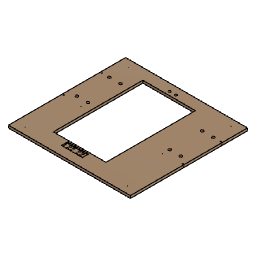
Underbase (Autodesk Fusion 360 design; units mm, degrees)
Autodesk Fusion 360 part; units mm, degrees
sketch "Sketch1" plane through (0, 0, 0) normal (0, 0, 1) x (1, 0, 0)
  line L0 (440, 422.75) -> (-440, 422.75)
  line L1 (-440, 422.75) -> (-440, -422.75)
  line L2 (-440, -422.75) -> (440, -422.75)
  line L3 (440, -422.75) -> (440, 422.75)
  line L4 (440, 422.75) -> (-440, -422.75) construction
  line L5 (-440, 422.75) -> (440, -422.75) construction
  line L6 (144, -302.75) -> (-236, -302.75)
  line L7 (-236, -302.75) -> (-236, 342.75)
  line L8 (-236, 342.75) -> (144, 342.75)
  line L9 (144, 342.75) -> (144, -302.75)
  line L10 (-295, 5.75) -> (-375, 5.75) construction
  line L11 (-375, 5.75) -> (-375, 240.75) construction
  line L12 (-375, 240.75) -> (-295, 240.75) construction
  line L13 (-295, 240.75) -> (-295, 5.75) construction
  line L14 (375, 5.75) -> (295, 5.75) construction
  line L15 (295, 5.75) -> (295, 240.75) construction
  line L16 (295, 240.75) -> (375, 240.75) construction
  line L17 (375, 240.75) -> (375, 5.75) construction
  line L18 (-46.5, -422.75) -> (-46.5, 422.75) construction
  line L19 (-91.5, -323.55) -> (-1.5, -323.55) construction
  line L20 (-1.5, -323.55) -> (-1.5, -347.55) construction
  line L21 (-1.5, -347.55) -> (-91.5, -347.55) construction
  line L22 (-91.5, -347.55) -> (-91.5, -323.55) construction
  line L23 (-26.5, -319.5853) -> (-26.5, -354.5853) construction
  line L24 (-66.5, -319.5853) -> (-66.5, -354.5853) construction
  circle A0 centre (-26.5, -323.55) radius 6.35
  circle A1 centre (-26.5, -347.55) radius 6.35
  circle A2 centre (-66.5, -323.55) radius 6.35
  circle A3 centre (-66.5, -347.55) radius 6.35
  circle A4 centre (-91.5, -323.55) radius 7.95
  circle A5 centre (-91.5, -347.55) radius 7.95
  circle A6 centre (-1.5, -323.55) radius 7.95
  circle A7 centre (-1.5, -347.55) radius 7.95
  circle A8 centre (-295, 5.75) radius 9.5
  circle A9 centre (-375, 5.75) radius 9.5
  circle A10 centre (-375, 240.75) radius 9.5
  circle A11 centre (-295, 240.75) radius 9.5
  circle A12 centre (295, 240.75) radius 9.5
  circle A13 centre (375, 240.75) radius 9.5
  circle A14 centre (375, 5.75) radius 9.5
  circle A15 centre (295, 5.75) radius 9.5
  line L25 (100, 370.25) -> (-50, 370.25) construction
  circle A16 centre (-69.5, 370.25) radius 7.95
  circle A17 centre (-23.5, 370.25) radius 7.95
  line L26 (-440, 240.75) -> (440, 240.75) construction
  line L27 (-429, 260) -> (-429, -100) construction
  line L28 (429, 260) -> (429, -90) construction
  circle A18 centre (429, 240.75) radius 3.5
  circle A19 centre (429, 240.75) radius 9.5
  circle A20 centre (429, -34.25) radius 3.5
  circle A21 centre (429, -34.25) radius 9.5
  circle A22 centre (-429, 240.75) radius 3.5
  circle A23 centre (-429, 240.75) radius 9.5
  circle A24 centre (-429, -34.25) radius 3.5
  circle A25 centre (-429, -34.25) radius 9.5
  circle A26 centre (-370, -372.75) radius 1.5
  circle A27 centre (370, -372.75) radius 1.5
  circle A28 centre (-370, 372.75) radius 1.5
  circle A29 centre (370, 372.75) radius 1.5
  circle A30 centre (295, -44.25) radius 1.5
  circle A31 centre (-295, -44.25) radius 1.5
  dimension "d1" = 880
  dimension "d2" = 845.5
  dimension "d3" = 380
  dimension "d4" = 645.5
  dimension "d5" = 120
  dimension "d7" = 80
  dimension "d8" = 235
  dimension "d9" = 235
  dimension "d10" = 80
  dimension "d11" = 65
  dimension "d12" = 65
  dimension "d13" = 182
  dimension "d14" = 182
  dimension "d16" = 90
  dimension "d17" = 24
  dimension "d18" = 45
  dimension "d19" = 40
  dimension "d20" = 12.7
  dimension "d21" = 12.7
  dimension "d22" = 12.7
  dimension "d23" = 12.7
  dimension "d24" = 15.9
  dimension "d25" = 15.9
  dimension "d26" = 15.9
  dimension "d27" = 15.9
  dimension "d29" = 20
  dimension "d30" = 75.2
  dimension "d31" = 19
  dimension "d32" = 19
  dimension "d33" = 19
  dimension "d34" = 19
  dimension "d35" = 19
  dimension "d36" = 19
  dimension "d37" = 19
  dimension "d38" = 19
  dimension "d39" = 52.5
  dimension "d40" = 15.9
  dimension "d41" = 15.9
  dimension "d42" = 23
  dimension "d43" = 23
  dimension "d44" = 11
  dimension "d45" = 11
  dimension "d46" = 7
  dimension "d47" = 19
  dimension "d48" = 7
  dimension "d49" = 19
  dimension "d50" = 275
  dimension "d51" = 7
  dimension "d52" = 19
  dimension "d53" = 7
  dimension "d54" = 275
  dimension "d55" = 19
  dimension "d66" = 296
  dimension "d67" = 486.5
  dimension "d84" = 3
  dimension "d85" = 3
  dimension "d86" = 3
  dimension "d87" = 3
  dimension "d88" = 3
  dimension "d89" = 3
  dimension "d90" = 70
  dimension "d91" = 70
  dimension "d92" = 70
  dimension "d93" = 70
  dimension "d94" = 50
  dimension "d95" = 50
  dimension "d96" = 50
  dimension "d97" = 50
  dimension "d98" = 50
  dimension "d99" = 50
  constraint perpendicular L0 L1
  constraint parallel L0 L2
  constraint parallel L1 L3
  constraint horizontal L0
  constraint coincident L4 origin
  constraint coincident L5 origin
  constraint horizontal L6
  constraint vertical L7
  constraint horizontal L8
  constraint vertical L9
  constraint horizontal L10
  constraint vertical L11
  constraint horizontal L12
  constraint vertical L13
  constraint horizontal L14
  constraint vertical L15
  constraint horizontal L16
  constraint vertical L17
  constraint coincident L2 L18.start
  constraint coincident L0 L18.end
  constraint perpendicular L0 L18
  constraint horizontal L19
  constraint vertical L20
  constraint horizontal L21
  constraint vertical L22
  constraint perpendicular L21 L23
  constraint perpendicular L21 L24
  constraint coincident L23 A0.centre
  constraint coincident L19 A0.centre
  constraint coincident L23 A1.centre
  constraint coincident L21 A1.centre
  constraint coincident L19 A2.centre
  constraint coincident L24 A2.centre
  constraint coincident L24 A3.centre
  constraint coincident L21 A3.centre
  constraint coincident L19.start L22.end
  constraint coincident L21.end L22.start
  constraint coincident L19.end L20.start
  constraint coincident L20.end L21.start
  constraint coincident L10.start L13.end
  constraint coincident L10.end L11.start
  constraint coincident L11.end L12.start
  constraint coincident L12.end L13.start
  constraint coincident L15.end L16.start
  constraint coincident L16.end L17.start
  constraint coincident L14.start L17.end
  constraint coincident L14.end L15.start
  constraint perpendicular L18 L25
  constraint coincident L25 A16.centre
  constraint coincident L25 A17.centre
  constraint coincident L1 L26.start
  constraint coincident L3 L26.end
  constraint perpendicular L3 L26
  constraint collinear L12 L26
  constraint perpendicular L26 L27
  constraint perpendicular L26 L28
  constraint coincident L26 A18.centre
  constraint coincident L28 A18.centre
  constraint concentric A18 A19
  constraint coincident L28 A20.centre
  constraint concentric A20 A21
  constraint coincident L27 A22.centre
  constraint coincident L26 A22.centre
  constraint concentric A22 A23
  constraint coincident L27 A24.centre
  constraint concentric A24 A25
  measures "d1" distance of L1.end L2.end
  measures "d2" distance of L0.end L1.end
  measures "d3" distance of L6.start L6.end
  measures "d4" distance of L6.start L8.end
  measures "d5" distance of L2 L6
  measures "d7" distance of L10.start L10.end
  measures "d8" distance of L10.start L12.end
  measures "d9" distance of L14.start L16.end
  measures "d10" distance of L14.start L14.end
  measures "d11" distance of L1 L11
  measures "d12" distance of L3 L17
  measures "d13" distance of L0 L12
  measures "d14" distance of L0 L16
  measures "d16" distance of L19.start L19.end
  measures "d17" distance of L19.start L21.end
  measures "d18" distance of L18 L20
  measures "d19" distance of L23 L24
  measures "d20" diameter of A0
  measures "d21" diameter of A1
  measures "d22" diameter of A2
  measures "d23" diameter of A3
  measures "d24" diameter of A4
  measures "d25" diameter of A5
  measures "d26" diameter of A6
  measures "d27" diameter of A7
  measures "d29" distance of L18 L23
  measures "d30" distance of L2 L21
  measures "d31" diameter of A8
  measures "d32" diameter of A9
  measures "d33" diameter of A10
  measures "d34" diameter of A11
  measures "d35" diameter of A12
  measures "d36" diameter of A13
  measures "d37" diameter of A14
  measures "d38" diameter of A15
  measures "d39" distance of L0 L25
  measures "d40" diameter of A16
  measures "d41" diameter of A17
  measures "d42" distance of L18 A17.centre
  measures "d43" distance of L18 A16.centre
  measures "d44" distance of L1 L27
  measures "d45" distance of L3 L28
  measures "d46" diameter of A18
  measures "d47" diameter of A19
  measures "d48" diameter of A20
  measures "d49" diameter of A21
  measures "d50" distance of A18.centre A20.centre
  measures "d51" diameter of A22
  measures "d52" diameter of A23
  measures "d53" diameter of A24
  measures "d54" distance of A22.centre A24.centre
  measures "d55" diameter of A25
  measures "d66" distance of L3 L9
  measures "d67" distance of L3 L18
  measures "d84" diameter of A26
  measures "d85" diameter of A27
  measures "d86" diameter of A28
  measures "d87" diameter of A29
  measures "d88" diameter of A30
  measures "d89" diameter of A31
  measures "d90" distance of L1 A26.centre
  measures "d91" distance of L3 A27.centre
  measures "d92" distance of L3 A29.centre
  measures "d93" distance of L1 A28.centre
  measures "d94" distance of L2 A26.centre
  measures "d95" distance of L2 A27.centre
  measures "d96" distance of L0 A29.centre
  measures "d97" distance of L0 A28.centre
  measures "d98" distance of L10.start A31.centre
  measures "d99" distance of L14.end A30.centre
extrude "Extrude1" add sketch "Sketch1" along normal blind 18 contours L0 L1 L2 L3 | A19 | A21 | A23 | A25
extrude "Extrude2" cut sketch "Sketch1" along normal blind 5 contours A19 | A21 | A23 | A25
sketch "Sketch2" plane through (0, 0, 18) normal (0, 0, 1) x (-1, 0, 0)
  circle A0 centre (-429, -240.75) radius 3.5
  circle A1 centre (23.5, -370.25) radius 7.95
  circle A2 centre (-429, 34.25) radius 3.5
  circle A3 centre (69.5, -370.25) radius 7.95
  circle A4 centre (429, -240.75) radius 3.5
  circle A5 centre (429, 34.25) radius 3.5
  circle A6 centre (295, -5.75) radius 9.5
  circle A7 centre (375, -240.75) radius 9.5
  circle A8 centre (295, -240.75) radius 9.5
  circle A9 centre (-295, -240.75) radius 9.5
  circle A10 centre (-375, -240.75) radius 9.5
  circle A11 centre (-375, -5.75) radius 9.5
  circle A12 centre (-295, -5.75) radius 9.5
  circle A13 centre (1.5, 347.55) radius 7.95
  circle A14 centre (1.5, 323.55) radius 7.95
  circle A15 centre (91.5, 347.55) radius 7.95
  circle A16 centre (91.5, 323.55) radius 7.95
  circle A17 centre (66.5, 347.55) radius 6.35
  circle A18 centre (66.5, 323.55) radius 6.35
  circle A19 centre (26.5, 347.55) radius 6.35
  circle A20 centre (26.5, 323.55) radius 6.35
  circle A21 centre (375, -5.75) radius 9.5
  line L0 (236, -342.75) -> (-144, -342.75)
  line L1 (-144, -342.75) -> (-144, 302.75)
  line L2 (-144, 302.75) -> (236, 302.75)
  line L3 (236, 302.75) -> (236, -342.75)
  line L4 (-440, 422.75) -> (-440, -422.75)
  line L5 (-440, -422.75) -> (440, -422.75)
  line L6 (440, -422.75) -> (440, 422.75)
  line L7 (440, 422.75) -> (-440, 422.75)
  line L8 (122, 313.05) -> (-29, 313.05)
  line L9 (-29, 313.05) -> (-29, 358.05)
  line L10 (-29, 358.05) -> (122, 358.05)
  line L11 (122, 358.05) -> (122, 313.05)
  line L12 (1.5, 323.55) -> (-29, 323.55) construction
  line L13 (91.5, 323.55) -> (122, 323.55) construction
  line L14 (91.5, 323.55) -> (91.5, 313.05) construction
  line L15 (91.5, 347.55) -> (91.5, 358.05) construction
  circle A22 centre (429, 34.25) radius 9.5
  circle A23 centre (370, -372.75) radius 1.5
  circle A24 centre (-370, 372.75) radius 1.5
  circle A25 centre (-370, -372.75) radius 1.5
  circle A26 centre (-295, 44.25) radius 1.5
  circle A27 centre (295, 44.25) radius 1.5
  circle A28 centre (370, 372.75) radius 1.5
  dimension "d62" = 151
  dimension "d63" = 45
  dimension "d72" = 46
  dimension "d73" = 65
  dimension "d74" = 11
  dimension "d75" = 80
  dimension "d76" = 40
  dimension "d77" = 65
  dimension "d78" = 80
  dimension "d79" = 380
  dimension "d80" = 645.5
  dimension "d81" = 296
  dimension "d82" = 80
  dimension "d83" = 64.7
  constraint horizontal L8
  constraint vertical L9
  constraint horizontal L10
  constraint vertical L11
  constraint coincident A14.centre L12.start
  constraint coincident L9 L12.end
  constraint perpendicular L9 L12
  constraint coincident A16.centre L13.start
  constraint coincident L11 L13.end
  constraint perpendicular L11 L13
  constraint equal L12 L13
  constraint coincident L8 L14.end
  constraint perpendicular L8 L14
  constraint coincident A15.centre L15.start
  constraint coincident L10 L15.end
  constraint perpendicular L10 L15
  constraint equal L14 L15
  measures "d62" distance of L8.start L8.end
  measures "d63" distance of L8.start L10.end
  measures "d72" distance of A1.centre A3.centre
  measures "d73" distance of A7.centre L6
  measures "d74" distance of A4.centre L6
  measures "d75" distance of A7.centre A8.centre
  measures "d76" vertical distance of A21.centre A5.centre
  measures "d77" distance of A10.centre L4
  measures "d78" distance of A9.centre A10.centre
  measures "d79" distance of L0.start L0.end
  measures "d80" distance of L0.end L1.end
  measures "d81" distance of L1 L4
  measures "d82" distance of L0 L5
  measures "d83" distance of L7 L10
extrude "Extrude4" cut sketch "Sketch2" against normal blind 8.5 contours L8 L9 L10 L11
equation "d20 = M5WasherClearance"
equation "d21 = M5WasherClearance"
equation "d22 = M5WasherClearance"
equation "d23 = M5WasherClearance"
equation "d24 = M6WasherClearance"
equation "d25 = M6WasherClearance"
equation "d26 = M6WasherClearance"
equation "d27 = M6WasherClearance"
equation "d31 = CrossDowelClearance"
equation "d32 = CrossDowelClearance"
equation "d33 = CrossDowelClearance"
equation "d34 = CrossDowelClearance"
equation "d35 = CrossDowelClearance"
equation "d36 = CrossDowelClearance"
equation "d37 = CrossDowelClearance"
equation "d38 = CrossDowelClearance"
equation "d40 = M6WasherClearance"
equation "d41 = M6WasherClearance"
equation "d46 = M6ClearHole"
equation "d47 = CrossDowelClearance"
equation "d48 = M6ClearHole"
equation "d49 = CrossDowelClearance"
equation "d51 = M6ClearHole"
equation "d52 = CrossDowelClearance"
equation "d53 = M6ClearHole"
equation "d55 = CrossDowelClearance"
equation "CrossDowelClearance = 19 mm"
equation "M6ClearHole = 7 mm"
equation "M6WasherClearance = 15.9 mm"
equation "M5WasherClearance = 12.7 mm"
equation "d91 = d90"
equation "d92 = d90"
equation "d93 = d90"
equation "d95 = d94"
equation "d96 = d94"
equation "d97 = d94"
equation "d98 = d94"
equation "d99 = d94"
named bodies: "Underbase"
